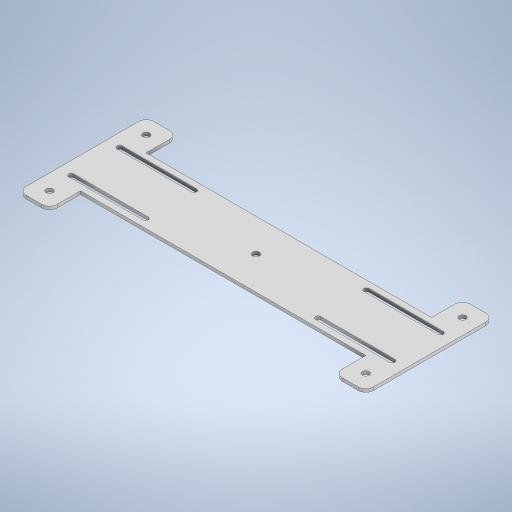
# Autodesk Inventor part: Motor Attachment 3.0
Saved by Autodesk Inventor 2024 (Build 280153000, 153)
## iProperties
Created: 2024-02-10
Part Number: Motor Attachment 3.0
Material: Generic
Document SubType Name: Modeling
Designer: olson
Density: 1 g/cm^3
Appearance: Default
Author: olson
Autodesk Inventor part; units mm, degrees
ref_plane "YZ Plane" through (0, 0, 0) normal (1, 0, 0) x (0, 1, 0)
ref_plane "XZ Plane" through (0, 0, 0) normal (0, 1, 0) x (-1, 0, 0)
ref_plane "XY Plane" through (0, 0, 0) normal (0, 0, 1) x (1, 0, 0)
sketch "Sketch1" plane through (0, 0, 0) normal (0, 1, 0) x (-1, 0, 0)
  line L0 (0, 0) -> (0, -42.4)
  line L1 (20, 0) -> (204, 0)
  line L2 (20, -42.4) -> (204, -42.4)
  line L3 (224, -42.4) -> (224, 0)
  line L4 (0, -42.4) -> (0, -62.4)
  line L5 (0, -62.4) -> (20, -62.4)
  line L6 (20, -62.4) -> (20, -42.4)
  line L7 (0, 0) -> (0, 20)
  line L8 (0, 20) -> (20, 20)
  line L9 (20, 20) -> (20, 0)
  line L10 (224, -42.4) -> (224, -62.4)
  line L11 (224, -62.4) -> (204, -62.4)
  line L12 (204, -62.4) -> (204, -42.4)
  line L13 (224, 0) -> (224, 20)
  line L14 (224, 20) -> (204, 20)
  line L15 (204, 20) -> (204, 0)
  circle A0 centre (10, -52.4) radius 2.125
  circle A1 centre (10, 10) radius 2.125
  circle A2 centre (214, -52.4) radius 2.125
  circle A3 centre (214, 10) radius 2.125
  circle A4 centre (112, -21.2) radius 2.125
  line L16 (0, -42.4) -> (0, -36.8)
  line L17 (0, -36.8) -> (8.4, -36.8)
  arc A5 (8.4, -35.2) -> (8.4, -38.4) centre (8.4, -36.8) ccw
  line L18 (0, 0) -> (0, -5.6)
  line L19 (0, -5.6) -> (8.4, -5.6)
  arc A6 (8.1881, -4.0141) -> (8.4, -7.2) centre (8.4, -5.6) ccw
  arc A7 (56.4, -38.4) -> (56.4, -35.2) centre (56.4, -36.8) ccw
  line L20 (8.4, -35.2) -> (56.4, -35.2)
  line L21 (56.4, -38.4) -> (8.4, -38.4)
  arc A8 (56.4, -7.2) -> (56.3995, -4) centre (56.4, -5.6) ccw
  line L22 (56.4, -7.2) -> (8.4, -7.2)
  line L23 (8.1881, -4.0141) -> (56.3995, -4)
  arc A9 (215.6, -38.4) -> (215.6, -35.2) centre (215.6, -36.8) ccw
  arc A10 (215.6, -7.2) -> (215.8119, -4.0141) centre (215.6, -5.6) ccw
  arc A11 (167.6, -35.2) -> (167.6, -38.4) centre (167.6, -36.8) ccw
  line L24 (215.6, -35.2) -> (167.6, -35.2)
  line L25 (167.6, -38.4) -> (215.6, -38.4)
  arc A12 (167.6005, -4) -> (167.6, -7.2) centre (167.6, -5.6) ccw
  line L26 (167.6, -7.2) -> (215.6, -7.2)
  line L27 (215.8119, -4.0141) -> (167.6005, -4)
  dimension "d1" = 42.4
  dimension "d2" = 224
  dimension "d3" = 224
  dimension "d4" = 20
  dimension "d5" = 20
  dimension "d6" = 20
  dimension "d7" = 20
  dimension "d8" = 20
  dimension "d9" = 20
  dimension "d10" = 4.25
  dimension "d11" = 4.25
  dimension "d12" = 4.25
  dimension "d13" = 4.25
  dimension "d14" = 4.25
  dimension "d15" = 5.6
  dimension "d16" = 8.4
  dimension "d17" = 3.2
  dimension "d18" = 5.6
  dimension "d19" = 3.2
  dimension "d23" = 3.2
  dimension "d28" = 3.2
  constraints: 56 end point, 16 point on circle, 13 centre point, 11 point on line, 5 perpendicular, 5 tangent, 4 coincident, 4 horizontal, 2 vertical
  measures "d1" distance of L0.start L0.end
  measures "d2" distance of L0.start L3.end
  measures "d3" distance of L0.end L3.start
  measures "d4" distance of L0.end L4.end
  measures "d5" distance of L4.end L5.end
  measures "d6" distance of L0.start L7.end
  measures "d7" distance of L3.start L10.end
  measures "d8" distance of L10.end L11.end
  measures "d9" distance of L3.end L13.end
  measures "d10" diameter of A0
  measures "d11" diameter of A1
  measures "d12" diameter of A2
  measures "d13" diameter of A3
  measures "d14" diameter of A4
  measures "d15" distance of L0.end L16.end
  measures "d16" distance of L16.end L17.end
  measures "d17" diameter of A5
  measures "d18" distance of L0.start L18.end
  measures "d19" diameter of A6
  measures "d23" diameter of A7
  measures "d28" diameter of A8
extrude "Extrusion1" add sketch "Sketch1" along normal blind 2
fillet "Fillet1" radius 5 8 edges at (0, 1, 20) (-20, 1, 20) (0, 1, -62.4) (-20, 1, -62.4) (-204, 1, -62.4) (-224, 1, -62.4) (-204, 1, 20) (-224, 1, 20)
body "Solid1"
